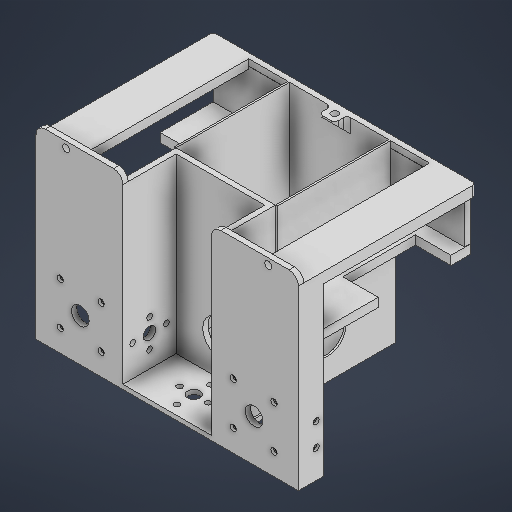
# Autodesk Inventor part: Base Shell Restart 2024 - Medium Drive Motors
Saved by Autodesk Inventor 2026.2 (Build 302298000, 298)
## iProperties
Created: 2024-09-23
Part Number: Base Shell Restart 2024 - Medium Drive Motors
Material: Generic
Document SubType Name: Modeling
Designer: Ethan
Density: 1 g/cm^3
Appearance: Default
Author: Ethan
Autodesk Inventor part; units mm, degrees
ref_plane "XZ Plane" through (0, 0, 0) normal (0, 1, 0) x (-1, 0, 0)
ref_plane "XY Plane" through (0, 0, 0) normal (0, 0, 1) x (1, 0, 0)
sketch "Sketch1" plane through (0, 0, 0) normal (0, 1, 0) x (-1, 0, 0)
  line L0 (74, -65.5068) -> (-74, -65.5068)
  line L1 (-74, -65.5068) -> (-74, 34.4932)
  line L2 (-74, 34.4932) -> (74, 34.4932)
  line L3 (74, 34.4932) -> (74, -65.5068)
  line L4 (-103.6, 0) -> (103.6, 0) construction
  line L5 (0, -85.5068) -> (0, 54.4932) construction
  point P0 (0, 0)
  dimension "d1" = 34.4932
  dimension "d2" = 148
  dimension "d219" = 65.5068
  dimension "d220" = 100
  constraints: 8 end point, 2 parallel, 1 horizontal, 1 perpendicular, 1 other
  measures "d1" distance between parallel lines of L4 L2
  measures "d2" distance between parallel lines of L3 L1
  measures "d219" distance between parallel lines of L0 L4
  measures "d220" distance between parallel lines of L0 L2
extrude "Base Bottom" add sketch "Sketch1" along normal blind 2.5
sketch "Sketch2" plane through (0, 0, 0) normal (0, 1, 0) x (-1, 0, 0)
  line L0 (74, 34.4932) -> (-74, 34.4932) projected
  line L1 (-74, 34.4932) -> (-74, -65.5068) projected
  line L2 (-74, -65.5068) -> (74, -65.5068) projected
  line L3 (74, -65.5068) -> (74, 34.4932) projected
  line L4 (71, -62.5068) -> (-71, -62.5068)
  line L5 (-71, -62.5068) -> (-71, 31.4932)
  line L6 (-71, 31.4932) -> (71, 31.4932)
  line L7 (71, 31.4932) -> (71, -62.5068)
  point P0 (0, 0)
  dimension "d10" = 3
  constraints: 8 end point, 3 other
  measures "d10" distance between parallel lines of L2 L4
extrude "Base Walls" add sketch "Sketch2" along normal blind 100
ref_plane "Front Inner Plane" through (71, 2.5, 31.4932) normal (0, 0, -1) x (-1, 0, 0)
ref_plane "Front Outer Plane" through (-74, 0, 34.4932) normal (0, 0, 1) x (1, 0, 0)
ref_plane "Right Inner Plane" through (-71, 2.5, -62.5068) normal (1, 0, 0) x (0, 0, -1)
ref_plane "Left Inner Plane" through (71, 2.5, 31.4932) normal (-1, 0, 0) x (0, 0, 1)
ref_plane "Back Inner Plane" through (-71, 2.5, -62.5068) normal (0, 0, 1) x (1, 0, 0)
ref_plane "Bottom Inner Plane" through (0, 2.5, 0) normal (0, 1, 0) x (1, 0, 0)
ref_plane "Top Plane" through (0, 100, 0) normal (0, 1, 0) x (1, 0, 0)
ref_plane "Left Outer Plane" through (74, 0, 34.4932) normal (1, 0, 0) x (0, 0, -1)
sketch "Right Side Nut Holes Sketch" plane through (-71, 2.5, -62.5068) normal (1, 0, 0) x (0, 0, -1)
  line L0 (-87, 26.5) -> (-87, 13.5) construction
  circle A0 centre (-87, 26.5) radius 3.235 construction
  line L1 (-88.6175, 29.3016) -> (-85.3825, 29.3016)
  line L2 (-85.3825, 29.3016) -> (-83.765, 26.5)
  line L3 (-83.765, 26.5) -> (-85.3825, 23.6984)
  line L4 (-85.3825, 23.6984) -> (-88.6175, 23.6984)
  line L5 (-88.6175, 23.6984) -> (-90.235, 26.5)
  line L6 (-90.235, 26.5) -> (-88.6175, 29.3016)
  line L7 (-90.235, 13.5) -> (-88.6175, 16.3016)
  line L8 (-88.6175, 16.3016) -> (-85.3825, 16.3016)
  line L9 (-85.3825, 16.3016) -> (-83.765, 13.5)
  line L10 (-83.765, 13.5) -> (-85.3825, 10.6984)
  line L11 (-85.3825, 10.6984) -> (-88.6175, 10.6984)
  line L12 (-88.6175, 10.6984) -> (-90.235, 13.5)
  line L13 (-97, -2.5) -> (-97, 97.5) projected
  line L14 (3, -2.5) -> (-97, -2.5) projected
  point P0 (-62.5068, -2.5)
  point P1 (-87, 20)
  dimension "d27" = 6.47
  dimension "d29" = 13
  dimension "d30" = 10
  dimension "d31" = 22.5
  constraints: 26 end point, 3 coincident, 2 horizontal, 1 midpoint, 1 parallel, 1 vertical, 29 other
  measures "d29" distance of L0.start L0.end
  measures "d30" distance between parallel lines of L13 L0
  measures "d31" distance from line of L14 point (-87, 20)
extrude "Right Side Nut Holes" cut sketch "Right Side Nut Holes Sketch" against normal blind 1.5
sketch "Sketch8" plane through (-71, 2.5, -62.5068) normal (1, 0, 0) x (0, 0, -1)
  circle A0 centre (-87, 26.5) radius 1.75
  circle A1 centre (-87, 13.5) radius 1.75
  point P0 (-62.5068, -2.5)
  point P1 (-87, 13.5)
  dimension "d34" = 3.5
  constraints: 2 centre point, 2 coincident, 1 equal radius
  measures "d34" diameter of A0
extrude "Right Side Bolt Holes" cut sketch "Sketch8" against normal through all
mirror "Left Side Nut and Bolt Holes" about plane through (0, 0, 0) normal (1, 0, 0) of "Right Side Nut Holes", "Right Side Bolt Holes"
sketch "Sketch9" plane through (-71, 2.5, -62.5068) normal (0, 0, 1) x (1, 0, 0)
  line L0 (71, 117.5) -> (71, -22.5) projected
  line L1 (115.5, 26.5) -> (115.5, 13.5) construction
  circle A0 centre (115.5, 26.5) radius 3.235 construction
  line L2 (112.6984, 24.8825) -> (112.6984, 28.1175)
  line L3 (112.6984, 28.1175) -> (115.5, 29.735)
  line L4 (115.5, 29.735) -> (118.3016, 28.1175)
  line L5 (118.3016, 28.1175) -> (118.3016, 24.8825)
  line L6 (118.3016, 24.8825) -> (115.5, 23.265)
  line L7 (115.5, 23.265) -> (112.6984, 24.8825)
  line L8 (112.6984, 11.8825) -> (112.6984, 15.1175)
  line L9 (112.6984, 15.1175) -> (115.5, 16.735)
  line L10 (115.5, 16.735) -> (118.3016, 15.1175)
  line L11 (118.3016, 15.1175) -> (118.3016, 11.8825)
  line L12 (118.3016, 11.8825) -> (115.5, 10.265)
  line L13 (115.5, 10.265) -> (112.6984, 11.8825)
  line L14 (145, -2.5) -> (-3, -2.5) projected
  line L15 (29.3016, 24.8825) -> (29.3016, 28.1175)
  line L16 (29.3016, 28.1175) -> (26.5, 29.735)
  line L17 (26.5, 29.735) -> (23.6984, 28.1175)
  line L18 (23.6984, 28.1175) -> (23.6984, 24.8825)
  line L19 (23.6984, 24.8825) -> (26.5, 23.265)
  line L20 (26.5, 23.265) -> (29.3016, 24.8825)
  line L21 (29.3016, 11.8825) -> (29.3016, 15.1175)
  line L22 (29.3016, 15.1175) -> (26.5, 16.735)
  line L23 (26.5, 16.735) -> (23.6984, 15.1175)
  line L24 (23.6984, 15.1175) -> (23.6984, 11.8825)
  line L25 (23.6984, 11.8825) -> (26.5, 10.265)
  line L26 (26.5, 10.265) -> (29.3016, 11.8825)
  point P0 (71, -2.5)
  point P1 (115.5, 20)
  point P2 (26.5, 26.5)
  point P3 (26.5, 13.5)
  dimension "d37" = 6.47
  dimension "d38" = 13
  dimension "d39" = 22.5
  dimension "d40" = 44.5
  constraints: 50 end point, 14 symmetric about line, 3 coincident, 3 vertical, 1 collinear, 1 midpoint, 29 other
  measures "d38" distance of L1.start L1.end
  measures "d39" distance from line of L14 point (115.5, 20)
  measures "d40" distance between parallel lines of L0 L1
extrude "Back Nut Holes" cut sketch "Sketch9" against normal blind 1.5
sketch "Sketch10" plane through (-71, 2.5, -62.5068) normal (0, 0, 1) x (1, 0, 0)
  circle A0 centre (115.5, 26.5) radius 1.75
  circle A1 centre (115.5, 13.5) radius 1.75
  circle A2 centre (26.5, 26.5) radius 1.75
  circle A3 centre (26.5, 13.5) radius 1.75
  point P0 (71, -2.5)
  dimension "d43" = 3.5
  constraints: 4 centre point, 4 coincident, 3 equal radius
  measures "d43" diameter of A0
extrude "Back Screw Holes" cut sketch "Sketch10" against normal through all
sketch "Sketch11" plane through (71, 2.5, 31.4932) normal (0, 0, -1) x (-1, 0, 0)
  line L0 (71, -22.5) -> (71, 117.5) construction
  line L1 (22, 21.5) -> (120, 21.5) construction
  circle A0 centre (22, 21.5) radius 5
  circle A1 centre (120, 21.5) radius 5
  line L2 (145, -2.5) -> (-3, -2.5) projected
  point P0 (71, -2.5)
  point P1 (71, 21.5)
  dimension "d46" = 24
  dimension "d47" = 10
  dimension "d48" = 98
  constraints: 2 centre point, 2 coincident, 2 end point, 1 equal radius, 1 horizontal, 1 midpoint, 1 point on line
  measures "d46" distance between parallel lines of L2 L1
  measures "d47" diameter of A1
  measures "d48" distance of L1.start L1.end
extrude "Front Peg Holes" cut sketch "Sketch11" against normal through all
sketch "Sketch12" plane through (71, 2.5, 31.4932) normal (0, 0, -1) x (-1, 0, 0)
  line L0 (145, 97.5) -> (-3, 97.5) projected
  line L1 (-3, 102.75) -> (145, 102.75)
  line L2 (-3, 102.75) -> (-3, 97.5)
  line L3 (145, 102.75) -> (145, 97.5)
  point P0 (71, -2.5)
  dimension "d59" = 5.25
  constraints: 6 end point, 2 perpendicular, 1 horizontal
  measures "d59" distance between parallel lines of L0 L1
extrude "Top Lid Mount" add sketch "Sketch12" against normal up to surface (3 mm away)
sketch "Sketch13" plane through (71, 2.5, 31.4932) normal (0, 0, -1) x (-1, 0, 0)
  circle A0 centre (10.75, 33.85) radius 3.235 construction
  line L0 (10.75, 33.85) -> (10.75, 9.85) construction
  circle A1 centre (10.75, 9.85) radius 3.235 construction
  line L1 (13.985, 33.85) -> (12.3675, 31.0484)
  line L2 (12.3675, 31.0484) -> (9.1325, 31.0484)
  line L3 (9.1325, 31.0484) -> (7.515, 33.85)
  line L4 (7.515, 33.85) -> (9.1325, 36.6516)
  line L5 (9.1325, 36.6516) -> (12.3675, 36.6516)
  line L6 (12.3675, 36.6516) -> (13.985, 33.85)
  line L7 (13.985, 9.85) -> (12.3675, 7.0484)
  line L8 (12.3675, 7.0484) -> (9.1325, 7.0484)
  line L9 (9.1325, 7.0484) -> (7.515, 9.85)
  line L10 (7.515, 9.85) -> (9.1325, 12.6516)
  line L11 (9.1325, 12.6516) -> (12.3675, 12.6516)
  line L12 (12.3675, 12.6516) -> (13.985, 9.85)
  line L13 (71, -22.5) -> (71, 117.5) construction
  line L14 (145, -2.5) -> (-3, -2.5) construction
  circle A2 centre (33.75, 33.85) radius 3.235 construction
  line L15 (33.75, 33.85) -> (33.75, 9.85) construction
  circle A3 centre (33.75, 9.85) radius 3.235 construction
  line L16 (36.985, 33.85) -> (35.3675, 31.0484)
  line L17 (35.3675, 31.0484) -> (32.1325, 31.0484)
  line L18 (32.1325, 31.0484) -> (30.515, 33.85)
  line L19 (30.515, 33.85) -> (32.1325, 36.6516)
  line L20 (32.1325, 36.6516) -> (35.3675, 36.6516)
  line L21 (35.3675, 36.6516) -> (36.985, 33.85)
  line L22 (36.985, 9.85) -> (35.3675, 7.0484)
  line L23 (35.3675, 7.0484) -> (32.1325, 7.0484)
  line L24 (32.1325, 7.0484) -> (30.515, 9.85)
  line L25 (30.515, 9.85) -> (32.1325, 12.6516)
  line L26 (32.1325, 12.6516) -> (35.3675, 12.6516)
  line L27 (35.3675, 12.6516) -> (36.985, 9.85)
  line L28 (128.015, 33.85) -> (129.6325, 31.0484)
  line L29 (129.6325, 31.0484) -> (132.8675, 31.0484)
  line L30 (132.8675, 31.0484) -> (134.485, 33.85)
  line L31 (134.485, 33.85) -> (132.8675, 36.6516)
  line L32 (132.8675, 36.6516) -> (129.6325, 36.6516)
  line L33 (129.6325, 36.6516) -> (128.015, 33.85)
  line L34 (128.015, 9.85) -> (129.6325, 7.0484)
  line L35 (129.6325, 7.0484) -> (132.8675, 7.0484)
  line L36 (132.8675, 7.0484) -> (134.485, 9.85)
  line L37 (134.485, 9.85) -> (132.8675, 12.6516)
  line L38 (132.8675, 12.6516) -> (129.6325, 12.6516)
  line L39 (129.6325, 12.6516) -> (128.015, 9.85)
  line L40 (111.485, 9.85) -> (109.8675, 12.6516)
  line L41 (106.6325, 31.0484) -> (109.8675, 31.0484)
  line L42 (109.8675, 31.0484) -> (111.485, 33.85)
  line L43 (105.015, 33.85) -> (106.6325, 31.0484)
  line L44 (105.015, 9.85) -> (106.6325, 7.0484)
  line L45 (109.8675, 7.0484) -> (111.485, 9.85)
  line L46 (111.485, 33.85) -> (109.8675, 36.6516)
  line L47 (109.8675, 36.6516) -> (106.6325, 36.6516)
  line L48 (106.6325, 36.6516) -> (105.015, 33.85)
  line L49 (106.6325, 12.6516) -> (105.015, 9.85)
  line L50 (109.8675, 12.6516) -> (106.6325, 12.6516)
  line L51 (106.6325, 7.0484) -> (109.8675, 7.0484)
  circle A4 centre (22, 21.5) radius 5 projected
  line L52 (10.75, 21.85) -> (33.75, 21.85) construction
  point P0 (71, -2.5)
  dimension "d52" = 6.47
  dimension "d51" = 24
  dimension "d53" = 60.25
  dimension "d57" = 23
  dimension "d210" = 0.35
  constraints: 102 end point, 24 symmetric about line, 6 coincident, 5 horizontal, 4 horizontal alignment, 2 midpoint, 2 vertical, 1 parallel, 60 other
  measures "d51" distance of L0.start L0.end
  measures "d53" distance between parallel lines of L0 L13
  measures "d57" distance between parallel lines of L0 L15
  measures "d210" distance from line of A4.centre L52
extrude "Front Nut Holes" cut sketch "Sketch13" against normal blind 1.5 contours L1 L2 L3 L4 L5 L6 | L7 L8 L9 L10 L11 L12 | L16 L17 L18 L19 L20 L21 | L22 L23 L24 L25 L26 L27 | L33 L32 L31 L30 L29 L28 | L39 L38 L37 L36 L35 L34 | L45 L51 L44 L49 L50 L40 | L43 L48 L47 L46 L42 L41
sketch "Sketch14" plane through (71, 2.5, 31.4932) normal (0, 0, -1) x (-1, 0, 0)
  circle A0 centre (10.75, 33.85) radius 1.75
  circle A1 centre (33.75, 33.85) radius 1.75
  circle A2 centre (33.75, 9.85) radius 1.75
  circle A3 centre (10.75, 9.85) radius 1.75
  line L0 (71, -22.5) -> (71, 117.5) construction
  circle A4 centre (131.25, 33.85) radius 1.75
  circle A5 centre (108.25, 33.85) radius 1.75
  circle A6 centre (108.25, 9.85) radius 1.75
  circle A7 centre (131.25, 9.85) radius 1.75
  point P0 (71, -2.5)
  dimension "d65" = 3.5
  constraints: 8 centre point, 4 coincident, 4 symmetric about line, 3 equal radius, 4 other
  measures "d65" diameter of A0
extrude "Front Screw Holes" cut sketch "Sketch14" against normal through all
sketch "Sketch16" plane through (0, 2.5, 0) normal (0, 1, 0) x (1, 0, 0)
  circle A0 centre (37.25, -24.4932) radius 3.235 construction
  line L0 (0, 85.5068) -> (0, -54.4932) construction
  line L1 (-71, -31.4932) -> (71, -31.4932) projected
  line L2 (35.6325, -27.2948) -> (34.015, -24.4932)
  line L3 (34.015, -24.4932) -> (35.6325, -21.6916)
  line L4 (35.6325, -21.6916) -> (38.8675, -21.6916)
  line L5 (38.8675, -21.6916) -> (40.485, -24.4932)
  line L6 (40.485, -24.4932) -> (38.8675, -27.2948)
  line L7 (38.8675, -27.2948) -> (35.6325, -27.2948)
  line L8 (-35.6325, -27.2948) -> (-34.015, -24.4932)
  line L9 (-34.015, -24.4932) -> (-35.6325, -21.6916)
  line L10 (-35.6325, -21.6916) -> (-38.8675, -21.6916)
  line L11 (-38.8675, -21.6916) -> (-40.485, -24.4932)
  line L12 (-40.485, -24.4932) -> (-38.8675, -27.2948)
  line L13 (-38.8675, -27.2948) -> (-35.6325, -27.2948)
  point P0 (0, 0)
  point P1 (-37.25, -24.4932)
  dimension "d80" = 6.47
  dimension "d78" = 37.25
  dimension "d79" = 7
  constraints: 24 end point, 7 symmetric about line, 1 coincident, 1 horizontal, 16 other
  measures "d78" distance from line of point (37.25, -24.493) L0
  measures "d79" distance from line of L1 point (37.25, -24.493)
extrude "Bottom Nut Holes" cut sketch "Sketch16" against normal blind 1.5
sketch "Sketch17" plane through (0, 2.5, 0) normal (0, 1, 0) x (1, 0, 0)
  circle A0 centre (37.25, -24.4932) radius 1.75
  circle A1 centre (-37.25, -24.4932) radius 1.75
  point P0 (0, 0)
  dimension "d83" = 3.5
  constraints: 2 centre point, 2 coincident, 1 equal radius
  measures "d83" diameter of A0
extrude "Bottom Screw Holes" cut sketch "Sketch17" against normal through all
sketch "Sketch15" plane through (71, 2.5, 31.4932) normal (0, 0, -1) x (-1, 0, 0)
  line L0 (145, 102.75) -> (-3, 102.75) construction
  line L1 (145, 102.75) -> (-3, 102.75) construction
  line L2 (71, -22.5) -> (71, 117.5) construction
  circle A0 centre (14, 99.25) radius 2
  line L3 (-32.6, 97.5) -> (174.6, 97.5) construction
  circle A1 centre (71, 99.25) radius 2
  circle A2 centre (128, 99.25) radius 2
  point P0 (71, -2.5)
  dimension "d69" = 1.75
  dimension "d70" = 57
  dimension "d71" = 4
  dimension "d72" = 1.75
  dimension "d73" = 1.75
  dimension "d74" = 57
  constraints: 3 centre point, 2 equal radius, 1 point on line
  measures "d69" distance from line of A0.centre L3
  measures "d70" distance from line of A0.centre L2
  measures "d71" diameter of A0
  measures "d72" distance from line of L3 A1.centre
  measures "d73" distance from line of L3 A2.centre
  measures "d74" distance from line of L2 A2.centre
extrude "Lid Holes" cut sketch "Sketch15" against normal up to surface (3 mm away)
sketch "Sketch18" plane through (0, 100, 0) normal (0, 1, 0) x (1, 0, 0)
  line L0 (-71, 62.5068) -> (71, 62.5068) construction
  line L1 (0, 85.5068) -> (0, -54.4932) construction
  line L2 (-4.5, 62.5068) -> (4.5, 62.5068)
  line L3 (4.5, 62.5068) -> (4.5, 55.5068)
  line L4 (4.5, 55.5068) -> (-4.5, 55.5068)
  line L5 (-4.5, 55.5068) -> (-4.5, 62.5068)
  circle A0 centre (0, 60.0068) radius 2
  point P0 (0, 0)
  dimension "d87" = 2.5
  dimension "d88" = 9
  dimension "d89" = 4
  dimension "d90" = 4.5
  constraints: 8 end point, 2 parallel, 2 point on line, 1 centre point, 1 horizontal, 1 perpendicular, 1 other
  measures "d87" distance from line of L0 A0.centre
  measures "d88" distance of L2.start L2.end
  measures "d89" diameter of A0
  measures "d90" distance from line of L4 A0.centre
extrude "Lid Insert - Top" add sketch "Sketch18" against normal blind 1
sketch "Sketch19" plane through (0, 0, 0) normal (1, 0, 0) x (0, 1, 0)
  line L0 (99, -62.5068) -> (99, -55.5068) projected
  line L1 (99, -55.5068) -> (92, -62.5068)
  line L2 (99, -62.5068) -> (92, -62.5068)
  point P0 (0, 0)
  dimension "d93" = 45
  constraints: 4 end point, 1 perpendicular
  measures "d93" angle of L0 L1
extrude "Lid Insert - Bottom" add sketch "Sketch19" along normal up to surface (9 mm away) from surface at -4.5
sketch "Sketch20" plane through (0, 99, -60.0068) normal (0, 1, 0) x (1, 0, 0)
  circle A0 centre (0, 0) radius 2 projected
  point P0 (0, -60.0068)
extrude "Lid Insert Hole" cut sketch "Sketch20" against normal up to surface surface through (0, 99, -55.5068) normal (0, -0.7071068, 0.7071068)
ref_plane "Weapon Motor Mount Center Plane" through (0, 0, 0) normal (1, 0, 0) x (0, 1, 0)
sketch "Sketch22" plane through (0, 2.5, 0) normal (0, 1, 0) x (1, 0, 0)
  line L0 (0, 85.5068) -> (0, -54.4932) construction
  line L1 (25, -34.4932) -> (-25, -34.4932) construction
  line L2 (-25, -34.4932) -> (-25, -4.4932)
  line L3 (-25, -4.4932) -> (25, -4.4932)
  line L4 (25, -4.4932) -> (25, -34.4932)
  line L5 (-74, -34.4932) -> (74, -34.4932) construction
  line L6 (-28, -1.4932) -> (-28, -34.4932)
  line L7 (28, -34.4932) -> (28, -1.4932)
  line L8 (28, -1.4932) -> (-28, -1.4932)
  line L9 (-28, -34.4932) -> (-25, -34.4932)
  line L10 (28, -34.4932) -> (25, -34.4932)
  point P0 (0, 0)
  dimension "d104" = 30
  dimension "d105" = 50
  dimension "d106" = 3
  dimension "d107" = 3
  dimension "d108" = 3
  constraints: 18 end point, 3 collinear, 3 parallel, 2 point on line, 1 horizontal, 1 perpendicular, 1 other
  measures "d104" distance of L3.end L1.start
  measures "d105" distance of L1.start L1.end
  measures "d106" distance between parallel lines of L2 L6
  measures "d107" distance between parallel lines of L4 L7
  measures "d108" distance between parallel lines of L8 L3
extrude "Weapon Motor Mount Walls" add sketch "Sketch22" along normal up to surface (97.5 mm away)
ref_plane "Left Motor Mount Plane" through (25, 2.5, 31.4932) normal (-1, 0, 0) x (0, 0, 1)
sketch "Left Motor Mount Screw Holes Sketch" plane through (25, 2.5, 31.4932) normal (-1, 0, 0) x (0, 0, 1)
  circle A0 centre (-12, 17.5) radius 3.5
  circle A1 centre (-12, 25.5) radius 1.625
  circle A2 centre (-12, 9.5) radius 1.625
  circle A3 centre (-2.5, 17.5) radius 1.625
  circle A4 centre (-21.5, 17.5) radius 1.625
  line L0 (-21.5, 17.5) -> (-2.5, 17.5) construction
  line L1 (-12, 25.5) -> (-12, 9.5) construction
  line L2 (3, 123.8) -> (3, -23.55) construction
  line L3 (-117, -2.5) -> (23, -2.5) construction
  point P0 (-31.4932, -2.5)
  dimension "d112" = 19
  dimension "d113" = 16
  dimension "d114" = 3.25
  dimension "d115" = 7
  dimension "d117" = 15
  dimension "d118" = 20
  constraints: 5 centre point, 5 coincident, 4 end point, 3 equal radius, 2 midpoint, 1 horizontal, 1 vertical
  measures "d112" distance of L0.start L0.end
  measures "d113" distance of L1.start L1.end
  measures "d114" diameter of A1
  measures "d115" diameter of A0
  measures "d117" distance from line of point (-12, 17.5) L2
  measures "d118" distance from line of L3 A0.centre
sketch "Sketch21" plane through (71, 2.5, 31.4932) normal (0, 0, -1) x (-1, 0, 0)
  line L0 (71, -22.5) -> (71, 117.5) construction
  line L1 (46, 102.75) -> (96, 102.75)
  line L2 (96, 102.75) -> (96, 0)
  line L3 (96, 0) -> (46, 0)
  line L4 (46, 0) -> (46, 102.75)
  line L5 (-32.6, 0) -> (174.6, 0) construction
  line L6 (145, 102.75) -> (-3, 102.75) construction
  line L7 (145, 102.75) -> (-3, 102.75) projected
  line L8 (46, 97.5) -> (46, 0) construction
  line L9 (46, 0) -> (46, 97.5) construction
  line L10 (96, 0) -> (96, 97.5) construction
  line L11 (96, 0) -> (96, 97.5) construction
  point P0 (71, -2.5)
  constraints: 8 end point, 4 collinear, 2 parallel, 1 horizontal, 1 perpendicular
extrude "Weapon Mount Front Opening" cut sketch "Sketch21" against normal up to surface (3 mm away)
extrude "Left Motor Mount Screw Holes" cut sketch "Left Motor Mount Screw Holes Sketch" against normal up to surface (3 mm away)
mirror "Right Motor Mount Screw Holes" about plane through (0, 0, 0) normal (1, 0, 0) of "Left Motor Mount Screw Holes"
sketch "Sketch34" plane through (0, 2.5, 0) normal (0, 1, 0) x (1, 0, 0)
  circle A0 centre (0, -19.4932) radius 3.5
  line L0 (0, -9.9932) -> (0, -28.9932) construction
  circle A1 centre (0, -9.9932) radius 1.625
  circle A2 centre (0, -28.9932) radius 1.625
  line L1 (-8, -19.4932) -> (8, -19.4932) construction
  circle A3 centre (8, -19.4932) radius 1.625
  circle A4 centre (-8, -19.4932) radius 1.625
  line L2 (0, 85.5068) -> (0, -54.4932) construction
  line L3 (25, -22.9932) -> (25, -15.9932) projected
  line L4 (0, -19.4932) -> (25, -19.4932) construction
  line L5 (25, -4.4932) -> (25, -34.4932) construction
  point P0 (0, 0)
  point P1 (0, 0)
  dimension "d197" = 7
  dimension "d198" = 3.25
  dimension "d199" = 19
  dimension "d200" = 16
  constraints: 6 end point, 5 centre point, 5 coincident, 3 equal radius, 3 midpoint, 2 point on line, 1 horizontal, 1 perpendicular, 1 vertical
  measures "d197" diameter of A0
  measures "d198" diameter of A1
  measures "d199" distance of L0.end L0.start
  measures "d200" distance of L1.start L1.end
extrude "Center Motor Mount Screw Holes" cut sketch "Sketch34" against normal up to surface (2.5 mm away)
sketch "Sketch25" plane through (71, 2.5, 31.4932) normal (-1, 0, 0) x (0, 0, 1)
  circle A0 centre (-21.5, 17.5) radius 1.55
  line L0 (3, 117.5) -> (3, -22.5) projected
  line L1 (-117, -2.5) -> (23, -2.5) projected
  point P0 (-31.4932, -2.5)
  point P1 (-21.5, 17.5)
  dimension "d128" = 3.1
  dimension "d129" = 24.5
  dimension "d130" = 20
  constraints: 1 centre point, 1 coincident
  measures "d128" diameter of A0
  measures "d129" distance from line of L0 point (-21.5, 17.5)
  measures "d130" distance from line of point (-21.5, 17.5) L1
extrude "Left Tool Access Hole" cut sketch "Sketch25" against normal up to surface (3 mm away)
mirror "Right Tool Access Hole" about plane through (0, 0, 0) normal (1, 0, 0) of "Left Tool Access Hole"
ref_plane "EDIT POSITION OF DRIVE MOTORS" through (74, 0, -35.4818) normal (0, 0, -1) x (-1, 0, 0)
fillet "Base Fillet Courners" radius 2 6 edges at (-4.5, 99.5, -55.5068) (4.5, 99.5, -55.5068) (-4.5, 96, -62.5068) (4.5, 96, -62.5068) (-74, 50, -65.5068) (74, 50, -65.5068)
fillet "Top Lid Fillet" radius 5.25 4 edges at (74, 105.25, 32.9932) (-74, 105.25, 32.9932) (-25, 105.25, 32.9932) (25, 105.25, 32.9932)
sketch "Sketch42" plane through (71, 2.5, 31.4932) normal (0, 0, -1) x (-1, 0, 0)
  line L0 (64.5, 97.5) -> (0, 97.5) projected
  line L1 (0, 97.5) -> (20, 97.5)
  line L2 (20, 97.5) -> (20, 92.5)
  line L3 (20, 92.5) -> (0, 92.5)
  line L4 (0, 92.5) -> (0, 97.5)
  line L5 (-1, 97.5) -> (143, 97.5) projected
  line L6 (122, 97.5) -> (142, 97.5)
  line L7 (142, 97.5) -> (142, 92.5)
  line L8 (142, 92.5) -> (122, 92.5)
  line L9 (122, 92.5) -> (122, 97.5)
  line L10 (99, 97.5) -> (99, 0) projected
  line L11 (43, 0) -> (43, 97.5) projected
  line L12 (0, 0) -> (0, 97.5) projected
  line L13 (142, 0) -> (142, 97.5) projected
  point P0 (71, -2.5)
  dimension "d235" = 5
  dimension "d236" = 5
  dimension "d237" = 20
  dimension "d238" = 20
  dimension "d255" = 0
  dimension "d256" = 0
  constraints: 16 end point, 4 parallel, 2 horizontal, 2 perpendicular, 1 point on line, 2 other
  measures "d235" distance of L1.end L2.end
  measures "d236" distance of L6.end L7.end
  measures "d237" distance between parallel lines of L2 L4
  measures "d238" distance between parallel lines of L7 L9
  measures "d255" distance between parallel lines of L4 L12
  measures "d256" distance between parallel lines of L13 L7
extrude "Servo Hangers" add sketch "Sketch42" along normal through all
sketch "Sketch43" plane through (-74, 0, -63.5068) normal (-1, 0, 0) x (0, 0, 1)
  line L0 (-2, 0) -> (-2, 100) projected
  line L1 (98, 0) -> (0, 0) projected
  line L2 (-2, 94) -> (84, 94)
  line L3 (84, 94) -> (84, 0)
  line L4 (84, 0) -> (-2, 0)
  line L5 (-2, 0) -> (-2, 94)
  line L6 (0, 100) -> (95, 100) projected
  circle A0 centre (88, 29) radius 1.75 projected
  point P0 (63.5068, 0)
  dimension "d241" = 6
  dimension "d242" = 4
  constraints: 8 end point, 2 parallel, 2 point on line, 1 horizontal, 1 perpendicular
  measures "d241" distance between parallel lines of L6 L2
  measures "d242" distance from line of A0.centre L3
extrude "Cut For Wheels 1" cut sketch "Sketch43" against normal blind 45 contours L0 L2 L3 L1 L4
sketch "Sketch45" plane through (74, 0, 34.4932) normal (1, 0, 0) x (0, 0, -1)
  line L0 (14, 2.5) -> (14, 94) projected
  line L1 (100, 0) -> (98, 0) projected
  line L2 (14, 94) -> (100, 94)
  line L3 (100, 94) -> (100, 0)
  line L4 (100, 0) -> (14, 0)
  line L5 (14, 0) -> (14, 94)
  line L6 (3, 100) -> (98, 100) projected
  circle A0 centre (10, 29) radius 1.75 projected
  point P0 (34.4932, 0)
  point P1 (13, 29.407)
  point P2 (13, 29.407)
  dimension "d245" = 6
  dimension "d248" = 4
  constraints: 8 end point, 2 parallel, 1 horizontal, 1 perpendicular, 1 other
  measures "d245" distance between parallel lines of L6 L2
extrude "Cut for Wheels 2" cut sketch "Sketch45" against normal blind 45 contours L0 L2 L3 L1 L4 L5
sketch "Sketch46" plane through (-25, 100, 4.4932) normal (0, 0, 1) x (1, 0, 0)
  circle A0 centre (25, -77.5) radius 10
  line L0 (50, 0) -> (0, 0) projected
  line L1 (50, -97.5) -> (0, -97.5) projected
  point P0 (25, -100)
  dimension "d251" = 20
  dimension "d259" = 20
  constraints: 1 centre point
  measures "d251" diameter of A0
  measures "d259" distance from line of L1 A0.centre
extrude "Hole for B.Motor Wire" cut sketch "Sketch46" against normal blind 10
sketch "Sketch48" plane through (71, 2.5, 31.4932) normal (0, 0, -1) x (-1, 0, 0)
  line L0 (0, 66.5) -> (42, 66.5)
  line L1 (42, 66.5) -> (42, 61.5)
  line L2 (42, 61.5) -> (0, 61.5)
  line L3 (0, 61.5) -> (0, 66.5)
  line L4 (0, 91.5) -> (0, 0) projected
  line L5 (-1, 91.5) -> (42, 91.5) projected
  line L6 (42, 91.5) -> (42, -2.5) projected
  point P0 (71, -2.5)
  point P1 (42, 64)
  dimension "d261" = 0
  dimension "d265" = 5
  dimension "d266" = 30
  dimension "d267" = 0
  constraints: 8 end point, 2 parallel, 1 horizontal, 1 midpoint, 1 perpendicular
  measures "d261" distance between parallel lines of L3 L4
  measures "d265" distance between parallel lines of L2 L0
  measures "d266" distance between parallel lines of L5 L2
  measures "d267" distance between parallel lines of L6 L1
extrude "Servo Hanger" add sketch "Sketch48" along normal blind 97.142 contours L0 L1 L2 L3
sketch "Sketch50" plane through (29, 69, 31.4932) normal (0, 1, 0) x (1, 0, 0)
  line L0 (0, 97) -> (0, 11) projected
  line L1 (43, 97) -> (-101, 97) projected
  line L2 (0, 93.8887) -> (41.7803, 93.8887)
  line L3 (41.7803, 93.8887) -> (41.7803, 97)
  line L4 (41.7803, 97) -> (0, 97)
  line L5 (0, 97) -> (0, 93.8887)
  point P0 (-29, 31.4932)
  constraints: 8 end point, 2 parallel, 2 point on line, 1 horizontal, 1 perpendicular
extrude "Extrusion46" add sketch "Sketch50" along normal blind 27.405
sketch "Sketch51" plane through (29, 69, 31.4932) normal (0, 1, 0) x (1, 0, 0)
  line L0 (22, 45) -> (42, 45)
  line L1 (42, 45) -> (42, 86)
  line L2 (42, 86) -> (22, 86)
  line L3 (22, 86) -> (22, 45)
  line L4 (42, 0) -> (42, 94) projected
  line L5 (1.25, 0) -> (39.75, 0) projected
  point P0 (-29, 31.4932)
  dimension "d274" = 20
  dimension "d275" = 0
  dimension "d276" = 41
  dimension "d277" = 45
  constraints: 8 end point, 2 parallel, 1 horizontal, 1 perpendicular
  measures "d274" distance between parallel lines of L1 L3
  measures "d275" distance between parallel lines of L4 L1
  measures "d276" distance between parallel lines of L2 L0
  measures "d277" distance between parallel lines of L5 L0
extrude "Cut for Servo" cut sketch "Sketch51" against normal blind 10
mirror "Mirror6" about plane through (0, 0, 0) normal (1, 0, 0) of "Servo Hanger"
mirror "Mirror7" about plane through (0, 0, 0) normal (1, 0, 0) of "Extrusion46"
sketch "Sketch53" plane through (0, 2.5, 0) normal (0, 1, 0) x (1, 0, 0)
  line L0 (-28, -1.4932) -> (28, -1.4932) projected
  line L1 (29, -20.4932) -> (29, 62.5068) projected
  line L2 (28, -1.4932) -> (29, -1.4932)
  line L3 (29, -1.4932) -> (29, 62.5068)
  line L4 (29, 62.5068) -> (28, 62.5068)
  line L5 (28, 62.5068) -> (28, -1.4932)
  point P0 (0, 0)
  constraints: 8 end point, 2 parallel, 1 horizontal, 1 perpendicular
extrude "Wall for Electronics" add sketch "Sketch53" along normal blind 97.5
mirror "Mirror9" about plane through (0, 0, 0) normal (1, 0, 0) of "Wall for Electronics"
sketch "Sketch54" plane through (29, 0, 34.4932) normal (1, 0, 0) x (0, 0, -1)
  circle A0 centre (61.7593, 22.4849) radius 10
  point P0 (34.4932, 0)
  dimension "d282" = 20
  constraints: 1 centre point
  measures "d282" diameter of A0
extrude "Extrusion50" cut sketch "Sketch54" against normal blind 5
mirror "Mirror10" about plane through (0, 0, 0) normal (1, 0, 0) of "Extrusion50"
sketch "Sketch57" plane through (29, 64, 31.4932) normal (0, -1, 0) x (1, 0, 0)
  circle A0 centre (37, -42) radius 1.75
  circle A1 centre (27.7, -42) radius 1.75
  circle A2 centre (37, -89) radius 1.75
  circle A3 centre (27.7, -89) radius 1.75
  line L0 (42, -11) -> (42, -45) projected
  line L1 (22, -45) -> (42, -45) projected
  line L2 (42, -86) -> (42, -97.142) projected
  line L3 (42, -86) -> (22, -86) projected
  point P0 (-29, -31.4932)
  dimension "d305" = 5
  dimension "d306" = 9.3
  dimension "d307" = 3.5
  dimension "d308" = 3.5
  dimension "d309" = 3
  dimension "d310" = 3
  dimension "d311" = 3.5
  dimension "d312" = 3.5
  dimension "d313" = 9.3
  dimension "d314" = 5
  dimension "d315" = 3
  dimension "d316" = 3
  constraints: 4 centre point
  measures "d305" distance from line of L0 A0.centre
  measures "d306" distance of A0.centre A1.centre
  measures "d307" diameter of A1
  measures "d308" diameter of A0
  measures "d309" distance from line of L1 A1.centre
  measures "d310" distance from line of L1 A0.centre
  measures "d311" diameter of A2
  measures "d312" diameter of A3
  measures "d313" distance of A3.centre A2.centre
  measures "d314" distance from line of L2 A2.centre
  measures "d315" distance from line of L3 A2.centre
  measures "d316" distance from line of L3 A3.centre
extrude "Servo Screw Holes" cut sketch "Sketch57" against normal blind 3
sketch "Sketch58" plane through (-71, 69, -65.6488) normal (0, 1, 0) x (1, 0, 0)
  line L0 (0, -86.142) -> (0, -3.142) projected
  line L1 (0, -74.153) -> (20, -74.153)
  line L2 (20, -74.153) -> (20, -33.153)
  line L3 (20, -33.153) -> (0, -33.153)
  line L4 (0, -33.153) -> (0, -74.153)
  line L5 (42, -86.142) -> (0, -86.142) projected
  line L6 (2.25, -97.142) -> (40.75, -97.142) projected
  point P0 (71, -65.6488)
  point P1 (0, -33.153)
  dimension "d322" = 22.989
  dimension "d323" = 41
  dimension "d339" = 20
  constraints: 8 end point, 2 parallel, 1 horizontal, 1 perpendicular, 1 point on line
  measures "d322" distance between parallel lines of L6 L1
  measures "d323" distance between parallel lines of L3 L1
  measures "d339" distance of L2.end L3.end
extrude "Cut for Servo 2" cut sketch "Sketch58" against normal blind 10
sketch "Sketch59" plane through (-71, 64, -65.6488) normal (0, -1, 0) x (1, 0, 0)
  circle A0 centre (5, 30.153) radius 1.75
  circle A1 centre (14.3, 30.153) radius 1.75
  circle A2 centre (5, 77.153) radius 1.75
  circle A3 centre (14.3, 77.153) radius 1.75
  line L0 (0, 74.153) -> (20, 74.153) projected
  line L1 (20, 33.153) -> (0, 33.153) projected
  line L2 (0, 33.153) -> (0, 0) projected
  line L3 (0, 86.142) -> (0, 74.153) projected
  point P0 (71, 65.6488)
  dimension "d324" = 3.5
  dimension "d325" = 3
  dimension "d326" = 3
  dimension "d327" = 3
  dimension "d328" = 3
  dimension "d329" = 3.5
  dimension "d330" = 3.5
  dimension "d331" = 3.5
  dimension "d335" = 9.3
  dimension "d336" = 9.3
  dimension "d337" = 5
  dimension "d338" = 5
  constraints: 4 centre point
  measures "d324" diameter of A0
  measures "d325" distance from line of L0 A2.centre
  measures "d326" distance from line of L0 A3.centre
  measures "d327" distance from line of L1 A0.centre
  measures "d328" distance from line of L1 A1.centre
  measures "d329" diameter of A1
  measures "d330" diameter of A2
  measures "d331" diameter of A3
  measures "d335" distance of A3.centre A2.centre
  measures "d336" distance of A1.centre A0.centre
  measures "d337" distance from line of L2 A0.centre
  measures "d338" distance from line of L3 A2.centre
extrude "Servo Screw Holes 2" cut sketch "Sketch59" against normal blind 3
equation "\"d72\" = d69"
equation "\"d73\" = d69"
equation "\"d74\" = d70"
equation "\"d90\" = 0.5 * d88"
equation "\"d106\" = d108"
equation "\"d107\" = d108"
body "Solid1"
